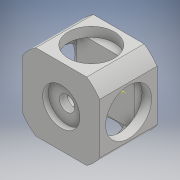
# Autodesk Inventor part: hub
Saved by Autodesk Inventor 2018 (Build 220112000, 112)
## iProperties
Created: 2018-11-06
Part Number: hub
Material: Generic
Document SubType Name: Modeling
Designer: HP
Density: 1 g/cm^3
Appearance: Default
Author: HP
Autodesk Inventor part; units mm, degrees
ref_plane "YZ Plane" through (0, 0, 0) normal (1, 0, 0) x (0, 1, 0)
ref_plane "XZ Plane" through (0, 0, 0) normal (0, 1, 0) x (-1, 0, 0)
ref_plane "XY Plane" through (0, 0, 0) normal (0, 0, 1) x (1, 0, 0)
sketch "Sketch1" plane through (0, 0, 0) normal (0, 1, 0) x (-1, 0, 0)
  line L0 (-66.3325, -100) -> (66.3325, -100)
  line L1 (100, -66.3325) -> (100, 66.3325)
  line L2 (66.3325, 100) -> (-66.3325, 100)
  line L3 (-100, 66.3325) -> (-100, -66.3325)
  line L4 (-100, -100) -> (100, 100) construction
  line L5 (100, -100) -> (-100, 100) construction
  arc A0 (100, 66.3325) -> (66.3325, 100) centre (0, 0) ccw
  arc A1 (66.3325, -100) -> (100, -66.3325) centre (0, 0) ccw
  arc A2 (-66.3325, 100) -> (-100, 66.3325) centre (0, 0) ccw
  arc A3 (-100, -66.3325) -> (-66.3325, -100) centre (0, 0) ccw
  line L6 (60, 75) -> (-60, 75)
  line L7 (-75, 60) -> (-75, -60)
  line L8 (-60, -75) -> (60, -75)
  line L9 (75, -60) -> (75, 60)
  line L10 (75, 75) -> (-75, -75) construction
  line L11 (-75, 75) -> (75, -75) construction
  arc A4 (75, 60) -> (60, 75) centre (60, 60) ccw
  arc A5 (60, -75) -> (75, -60) centre (60, -60) ccw
  arc A6 (-75, -60) -> (-60, -75) centre (-60, -60) ccw
  arc A7 (-60, 75) -> (-75, 60) centre (-60, 60) ccw
  dimension "d0" = 200
  dimension "d1" = 200
  dimension "d3" = 150
  dimension "d4" = 150
  dimension "d5" = 15
  constraints: 24 end point, 16 point on circle, 8 centre point, 8 point on line, 8 tangent, 4 midpoint, 4 parallel, 3 equal radius, 2 horizontal, 2 perpendicular, 1 coincident
  measures "d0" distance of L5.end L4.end
  measures "d1" distance of L4.end L5.start
  measures "d3" distance of L11.end L10.end
  measures "d4" distance of L10.end L11.start
  measures "d5" radius of A4
extrude "Extrusion1" add sketch "Sketch1" along normal mid plane 150
sketch "Sketch2" plane through (0, 75, 0) normal (0, 1, 0) x (1, 0, 0)
  line L0 (66.3325, 100) -> (-66.3325, 100)
  line L1 (-100, 100) -> (-100, -66.3325)
  line L2 (-100, -100) -> (100, -100)
  line L3 (100, -66.3325) -> (100, 100)
  line L4 (100, 100) -> (-100, -100) construction
  line L5 (-100, 100) -> (100, -100) construction
  arc A0 (-100, -66.3325) -> (-66.3325, -100) centre (0, 0) ccw
  arc A1 (-66.3325, 100) -> (-100, 66.3325) centre (0, 0) ccw
  arc A2 (66.3325, -100) -> (100, -66.3325) centre (0, 0) ccw
  arc A3 (100, 66.3325) -> (66.3325, 100) centre (0, 0) ccw
  dimension "d8" = 200
  dimension "d9" = 200
  constraints: 12 end point, 8 point on circle, 4 centre point, 4 point on line, 2 midpoint, 2 parallel, 1 coincident, 1 horizontal, 1 perpendicular
  measures "d8" distance of L2.end L2.start
  measures "d9" distance of L2.start L1.start
extrude "Extrusion2" add sketch "Sketch2" against normal blind 35
hole "Hole1" at (0, 75, 0) direction (0, -1, 0) diameter 40 end through all
sketch "Sketch3" plane through (-66.3325, -75, 100) normal (0, 0, 1) x (1, 0, 0)
  line L0 (46.3325, 185) -> (86.3325, 185)
  line L1 (86.3325, 185) -> (86.3325, 135)
  line L2 (46.3325, 115) -> (46.3325, 185)
  line L3 (132.665, 150) -> (0, 150) projected
  line L4 (46.3325, 185) -> (86.3325, 115) construction
  line L5 (86.3325, 185) -> (46.3325, 115) construction
  line L6 (86.3325, 115) -> (86.3325, 150) projected
  line L7 (46.3325, 165) -> (86.3325, 165)
  line L8 (86.3325, 165) -> (86.3325, 135)
  line L9 (46.3325, 135) -> (46.3325, 165)
  line L10 (46.3325, 165) -> (86.3325, 135) construction
  line L11 (86.3325, 165) -> (46.3325, 135) construction
  line L12 (86.3325, 135) -> (66.3325, 78.4315)
  line L13 (86.3325, 115) -> (79.2614, 115)
  line L14 (66.3325, 115) -> (46.3325, 115)
  line L15 (86.3325, 135) -> (74.9039, 135)
  line L16 (66.3325, 135) -> (46.3325, 135)
  line L17 (66.3325, 75) -> (66.3325, 115)
  circle A0 centre (66.3325, 78.4315) radius 60
  point P0 (66.3325, 150)
  dimension "d21" = 40
  dimension "d22" = 70
  dimension "d23" = 30
  dimension "d24" = 60
  constraints: 32 end point, 6 parallel, 4 point on line, 3 midpoint, 2 horizontal, 2 perpendicular, 1 coincident, 1 vertical, 3 other
  measures "d21" distance of L4.end L2.start
  measures "d22" distance of L0.end L4.end
  measures "d23" distance of L1.end L7.end
  measures "d24" distance of L1.end L12.end
extrude "Extrusion3" cut sketch "Sketch3" against normal blind 25 contours A0 L12 L17 L14 L2 | L2 L14 L17 L12 L13 L6 A0 | L6 L13 L12
mirror "Mirror1" about plane through (0, 0, 0) normal (0, 0, 1) of "Extrusion3"
sketch "Sketch4" plane through (-100, -75, -66.3325) normal (-1, 0, 0) x (0, 0, 1)
  line L0 (86.3325, 115) -> (86.3325, 150) projected
  line L1 (46.3325, 185) -> (86.3325, 185)
  line L2 (86.3325, 185) -> (86.3325, 132.5)
  line L3 (46.3325, 115) -> (46.3325, 185)
  line L4 (46.3325, 150) -> (86.3325, 150) projected
  line L5 (46.3325, 185) -> (86.3325, 115) construction
  line L6 (86.3325, 185) -> (46.3325, 115) construction
  line L7 (46.3325, 167.5) -> (86.3325, 167.5)
  line L8 (86.3325, 167.5) -> (86.3325, 132.5)
  line L9 (46.3325, 132.5) -> (46.3325, 167.5)
  line L10 (46.3325, 167.5) -> (86.3325, 132.5) construction
  line L11 (86.3325, 167.5) -> (46.3325, 132.5) construction
  line L12 (66.3325, 75) -> (66.3325, 115)
  line L13 (86.3325, 132.5) -> (66.3325, 75.9315)
  line L14 (86.3325, 132.5) -> (76.3325, 132.5)
  line L15 (56.3325, 132.5) -> (46.3325, 132.5)
  line L16 (66.3325, 115) -> (46.3325, 115)
  circle A0 centre (66.3325, 75.9315) radius 60
  point P0 (66.3325, 150)
  dimension "d27" = 60
  constraints: 30 end point, 5 parallel, 4 midpoint, 4 point on line, 2 horizontal, 2 perpendicular, 1 coincident, 1 vertical, 3 other
  measures "d27" distance of L2.end L13.end
extrude "Extrusion4" cut sketch "Sketch4" against normal blind 25 contours A0 L3 L16 L12 L13 | L13 L12 L16 L3 A0
mirror "Mirror2" about plane through (0, 0, 0) normal (1, 0, 0) of "Extrusion4"
sketch "Sketch5" plane through (0, 0, 0) normal (1, 0, 0) x (0, 1, 0)
  point P0 (0, 0)
sketch "Sketch6" plane through (0, -75, 0) normal (0, -1, 0) x (1, 0, 0)
  line L0 (-60, -75) -> (60, -75)
  line L1 (75, -60) -> (75, 60)
  line L2 (60, 75) -> (-60, 75)
  line L3 (-75, 60) -> (-75, -60)
  line L4 (-75, -75) -> (75, 75) construction
  line L5 (75, -75) -> (-75, 75) construction
  arc A0 (75, 60) -> (60, 75) centre (60, 60) ccw
  arc A1 (60, -75) -> (75, -60) centre (60, -60) ccw
  arc A2 (-75, -60) -> (-60, -75) centre (-60, -60) ccw
  arc A3 (-60, 75) -> (-75, 60) centre (-60, 60) ccw
  point P0 (0, 0)
  dimension "d21" = 40
  dimension "d30" = 150
  dimension "d31" = 150
  dimension "d32" = 15
  constraints: 12 end point, 8 point on circle, 8 point on line, 8 tangent, 4 centre point, 3 equal radius, 2 midpoint, 2 parallel, 1 horizontal, 1 perpendicular
  measures "d30" distance of L5.end L4.end
  measures "d31" distance of L4.end L5.start
  measures "d32" radius of A0
extrude "Extrusion5" add sketch "Sketch6" against normal blind 35
hole "Hole2" at (0, -75, 0) direction (0, 1, 0) diameter 40 end through all
sketch "Sketch7" plane through (0, 0, 0) normal (0, 0, 1) x (1, 0, 0)
  line L0 (47.5683, 40) -> (-47.5683, 40) projected
  line L1 (66.3325, 75) -> (-66.3325, 75) projected
  point P0 (0, 0)
  point P1 (47.5683, 75)
  constraints: 1 point on line
sketch "Sketch8" plane through (0, 75, 0) normal (0, 1, 0) x (1, 0, 0)
  circle A0 centre (0, 0) radius 48.6322
  constraints: 1 centre point, 1 coincident
extrude "Extrusion6" cut sketch "Sketch8" against normal blind 15
mirror "Mirror3" about plane through (0, 0, 0) normal (0, 1, 0) of "Extrusion6"
sketch "Sketch9" plane through (0, 0, 0) normal (0, 1, 0) x (-1, 0, 0)
  circle A0 centre (0, 0) radius 20
  constraints: 1 centre point, 1 coincident
body "Solid1"
